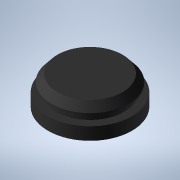
# Autodesk Inventor part: 0000-00168553(2)
Saved by Autodesk Inventor 2021 (Build 250183000, 183)
## iProperties
Created: 2025-08-26
Part Number: 0000-00168553(2)
Material: Generic
Catalog Web Link: www.cadenas.de
Description: Plug AX 2.0-Plug AX 2.0
Vendor: RITTAL
Document SubType Name: Modeling
Designer: psAdmin
Manufacturer: RITTAL
Mass: 1.80695 g
Surface Area: 10.6409 cm^2
Volume: 1.80695 cm^3
Density: 1 g/cm^3
Appearance: PSOLRGB-176-176-176
Category: PARTsolutions
Company: RITTAL
Title: 0000-00168553(2)
Author: Cadenas PARTsolutions
Comments: Plug AX 2.0
PSOL_IDENT_0: {$CADENAS_DATA/23d-libs/rittal/schaltschranksys/kompakt_schaltschr/parts_ae_2_0/plug_ax_2_0.prj},189
PSOL_IDENT_1: {VTYP=3D},{NB=0000-00168553(2)},{LINA=0000-00168553(2)},{NN=Plug AX 2.0},{DATE=20.08.2024 09:27:53}
PSOL_IDENT_2: ,{GEOMDATE=04.09.2019 09:18:26},{VERSION=},{LINEID=10},{WBVAR=DETAIL},{WBNUMERIC=DETAIL}  {NB=0000-0
PSOL_IDENT_3: 0168553(2)},{LINA=0000-00168553(2)},{KT=DUMMY},{BEST=0000-00168553},{DETAIL=2}
NB: 0000-00168553(2)
NN: Plug AX 2.0
NT: Plug AX 2.0
NBSYN: $BEST.($DETAIL.)
LINA: 0000-00168553(2)
CATALOG: Rittal
BEST: 0000-00168553
DETAIL: niedrig
SUPPLIER: RITTAL
ARTICLENO: 0000-00168553(2)
BOMINFO: 0000-00168553(2)
CREATOR: CADENAS GmbH
Autodesk Inventor part; units mm, degrees
sketch "Sketch_1" plane through (0, 0, 0) normal (0, 0, 1) x (1, 0, 0)
  line L0 (0, -3) -> (0, 3.85)
  line L1 (0, 3.85) -> (7.75, 3.85)
  line L2 (7.75, 3.85) -> (9.15, 2.1106)
  line L3 (9.15, 2.1106) -> (9.15, 1.7)
  line L4 (9.15, 1.7) -> (8.15, 1.3)
  line L5 (8.15, 1.3) -> (8.15, 0)
  line L6 (8.15, 0) -> (10, 0)
  line L7 (10, 0) -> (10, -3)
  line L8 (10, -3) -> (0, -3)
  line L9 (0, -3) -> (0, 3.85)
  constraints: 20 end point
revolve "Revolution1" add sketch "Sketch_1" angle 360 about axis through (0, -3, 0) along (0, -1, 0)
ref_plane "P1_XY" through (0, 0, 0) normal (0, 1, 0) x (1, 0, 0)
ref_plane "P1_YZ" through (0, 0, 0) normal (1, 0, 0) x (0, 0, -1)
ref_plane "P1_ZX" through (0, 0, 0) normal (0, 0, -1) x (0, 1, 0)
body "Solid1"
